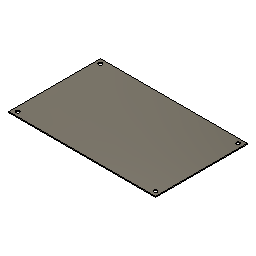
controller_final v10 (Autodesk Fusion 360 archive; units mm, degrees)
design "btt_octopus_footprint"
Autodesk Fusion 360 part; units mm, degrees
sketch "Sketch1" plane through (0, 0, 0) normal (0, 1, 0) x (1, 0, 0)
  line L0 (0, 0) -> (150, 0)
  line L1 (150, 0) -> (150, 90)
  line L2 (150, 90) -> (0, 90)
  line L3 (0, 90) -> (0, 0)
  circle A0 centre (0, 90) radius 2
  circle A1 centre (0, 0) radius 2
  circle A2 centre (150, 0) radius 2
  circle A3 centre (150, 90) radius 2
  line L4 (-5, -5) -> (155, -5)
  line L5 (155, -5) -> (155, 95)
  line L6 (155, 95) -> (-5, 95)
  line L7 (-5, 95) -> (-5, -5)
  dimension "d1" = 150
  dimension "d2" = 90
  dimension "d3" = 5
  dimension "d4" = 4
  constraint horizontal L0
  constraint vertical L1
  constraint horizontal L2
  constraint vertical L3
  constraint coincident L0.start L3.end
  constraint coincident L2.end L3.start
  constraint coincident L0.end L1.start
  constraint coincident L1.end L2.start
  constraint equal A0 A3
  constraint equal A0 A1
  constraint equal A1 A2
  measures "d1" distance of L0.start L0.end
  measures "d2" distance of L0.end L1.end
  measures "d4" diameter of A0
extrude "Extrude1" add sketch "Sketch1" along normal blind 1 contours L0 L1 L2 L3 A0 A1 A2 A3 | L4 L5 L6 L7
